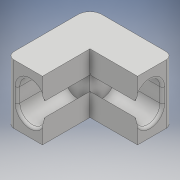
# Autodesk Inventor part: Gate Corner V5
Saved by Autodesk Inventor 2017 (Build 210142000, 142)
## iProperties
Created: 2018-11-10
Part Number: Gate Corner V5
Material: Generic
Document SubType Name: Modeling
Designer: djenl
Density: 1 g/cm^3
Appearance: Default
Author: djenl
Autodesk Inventor part; units mm, degrees
ref_plane "YZ Plane" through (0, 0, 0) normal (1, 0, 0) x (0, 1, 0)
ref_plane "XZ Plane" through (0, 0, 0) normal (0, 1, 0) x (-1, 0, 0)
ref_plane "XY Plane" through (0, 0, 0) normal (0, 0, 1) x (1, 0, 0)
sketch "Sketch1" plane through (0, 0, 0) normal (0, 0, 1) x (1, 0, 0)
  line L0 (0, 0) -> (15, 0)
  line L1 (15, 0) -> (15, -35)
  line L2 (15, -35) -> (0, -35)
  line L3 (0, -35) -> (0, 0)
  line L4 (0, 0) -> (35, 0)
  line L5 (35, 0) -> (35, -15)
  line L6 (35, -15) -> (0, -15)
  line L7 (0, -15) -> (0, 0)
  dimension "d0" = 15
  dimension "d1" = 35
  dimension "d2" = 35
  dimension "d3" = 15
  constraints: 16 end point, 4 parallel, 2 horizontal, 2 perpendicular
  measures "d0" distance of L1.end L2.end
  measures "d1" distance of L0.end L1.end
  measures "d2" distance of L5.end L6.end
  measures "d3" distance of L4.end L5.end
extrude "Extrusion1" add sketch "Sketch1" along normal blind 25
sketch "Sketch15" plane through (35, -15, 0) normal (1, 0, 0) x (0, 0, -1)
  line L0 (0, 0) -> (-25, 0) construction
  line L1 (0, 0) -> (0, 15) construction
  line L2 (-25, 0) -> (0, 0) construction
  line L3 (0, 0) -> (0, 10.4) construction
  line L4 (0, 10.4) -> (-25, 10.4) construction
  line L5 (-25, 10.4) -> (-25, 0) construction
  line L6 (-20.7, 0) -> (-4.3, 0) construction
  line L7 (-4.3, 0) -> (-4.3, 10.4) construction
  line L8 (-4.3, 10.4) -> (-20.7, 10.4) construction
  line L9 (-20.7, 10.4) -> (-20.7, 0) construction
  line L10 (-20.7, 0) -> (-4.3, 10.4) construction
  line L11 (-4.3, 0) -> (-20.7, 10.4) construction
  circle A0 centre (-15.5, 5.2) radius 5.2
  circle A1 centre (-9.5, 5.2) radius 5.2
  line L12 (-15.5, 0) -> (-9.5, 0)
  line L13 (-9.5, 0) -> (-9.5, 10.4)
  line L14 (-9.5, 10.4) -> (-15.5, 10.4)
  line L15 (-15.5, 10.4) -> (-15.5, 0)
  line L16 (-15.5, 0) -> (-9.5, 10.4) construction
  line L17 (-9.5, 0) -> (-15.5, 10.4) construction
  point P0 (-12.5, 5.2)
  dimension "d58" = 10.4
  dimension "d59" = 16.4
  dimension "d60" = 10.4
  constraints: 32 end point, 6 parallel, 5 horizontal, 4 midpoint, 3 perpendicular, 3 point on line, 3 tangent, 1 centre point, 1 vertical, 1 vertical alignment, 2 other
  measures "d58" distance of L3.end L2.end
  measures "d59" distance of L8.end L7.end
  measures "d60" distance of L6.end L7.end
extrude "Extrusion9" cut sketch "Sketch15" against normal blind 20
sketch "Sketch16" plane through (0, -35, 0) normal (0, -1, 0) x (1, 0, 0)
  line L0 (15, 25) -> (15, 15.5) construction
  line L1 (35, 0) -> (0, 0) construction
  line L2 (15, 25) -> (4.5, 25) construction
  line L3 (4.5, 25) -> (4.5, 0) construction
  line L4 (4.5, 0) -> (15, 0) construction
  line L5 (15, 0) -> (15, 25) construction
  line L6 (4.5, 20.75) -> (15, 20.75) construction
  line L7 (15, 20.75) -> (15, 4.25) construction
  line L8 (15, 4.25) -> (4.5, 4.25) construction
  line L9 (4.5, 4.25) -> (4.5, 20.75) construction
  line L10 (4.5, 20.75) -> (15, 4.25) construction
  line L11 (15, 20.75) -> (4.5, 4.25) construction
  circle A0 centre (9.75, 15.5) radius 5.25
  circle A1 centre (9.75, 9.5) radius 5.25
  line L12 (15, 15.5) -> (15, 9.5) projected
  line L13 (4.5, 15.5) -> (15, 15.5)
  line L14 (15, 15.5) -> (15, 9.5)
  line L15 (15, 9.5) -> (4.5, 9.5)
  line L16 (4.5, 9.5) -> (4.5, 15.5)
  line L17 (4.5, 15.5) -> (15, 9.5) construction
  line L18 (15, 15.5) -> (4.5, 9.5) construction
  point P0 (9.75, 12.5)
  dimension "d63" = 10.5
  dimension "d64" = 10.5
  dimension "d65" = 16.5
  constraints: 33 end point, 6 parallel, 4 horizontal, 4 midpoint, 3 perpendicular, 3 tangent, 2 vertical, 1 centre point, 1 horizontal alignment, 1 point on line, 2 other
  measures "d63" distance of L4.end L3.end
  measures "d64" distance of L7.end L8.end
  measures "d65" distance of L6.end L7.end
extrude "Extrusion10" cut sketch "Sketch16" against normal blind 20
fillet "Fillet10" radius 1 6 edges at (4.5, -35, 12.5) (9.75, -35, 4.25) (9.75, -35, 20.75) (35, -4.6, 12.5) (35, -9.8, 4.3) (35, -9.8, 20.7)
fillet "Fillet11" radius 5 1 edges at (0, 0, 12.5)
fillet "Fillet12" radius 3 2 edges at (0, -35, 12.5) (35, 0, 12.5)
body "Solid1"
